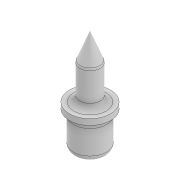
# Autodesk Inventor part: Punta calibración 2
Saved by Autodesk Inventor 2022 (Build 260153000, 153)
## iProperties
Created: 2022-11-17
Part Number: Punta calibración 2
Material: Generic
Document SubType Name: Modeling
Designer: ADMIN
Density: 1 g/cm^3
Appearance: Default
Author: ADMIN
## iProperties of the stored document Punta calibración 2_3DPrint.ipt
Created: 2022-11-17
Part Number: Punta calibración 2_3DPrint
Material: Generic
Document SubType Name: Modeling
Designer: ADMIN
Density: 1 g/cm^3
Appearance: Default
Author: ADMIN
Autodesk Inventor part; units mm, degrees
ref_plane "YZ Plane" through (0, 0, 0) normal (1, 0, 0) x (0, 1, 0)
ref_plane "XZ Plane" through (0, 0, 0) normal (0, 1, 0) x (-1, 0, 0)
ref_plane "XY Plane" through (0, 0, 0) normal (0, 0, 1) x (1, 0, 0)
sketch "Sketch1" plane through (0, 0, 0) normal (0, 1, 0) x (-1, 0, 0)
  circle A0 centre (0, 0) radius 5.6
  dimension "d0" = 11.2
  constraints: 1 centre point, 1 coincident
  measures "d0" diameter of A0
extrude "Extrusion1" add sketch "Sketch1" along normal blind 12
fillet "Fillet1" radius 2 1 edges at (5.6, 0, 0)
sketch "Sketch2" plane through (0, 12, 0) normal (0, 1, 0) x (1, 0, 0)
  circle A0 centre (0, 0) radius 7
  dimension "d4" = 14
  constraints: 1 centre point, 1 coincident
  measures "d4" diameter of A0
extrude "Extrusion2" add sketch "Sketch2" along normal blind 2
sketch "Sketch3" plane through (0, 0, 0) normal (1, 0, 0) x (0, 1, 0)
  line L0 (14, -7) -> (14, 7) projected
  line L1 (12, -7) -> (12, 7) projected
  line L2 (14, 0) -> (35, 0)
  line L3 (35, 0) -> (25.9829, -3.4613)
  line L4 (25.9829, -3.4613) -> (14, -3.4613)
  point P0 (0, 0)
  dimension "d7" = 21
  dimension "d8" = 21
  constraints: 6 end point, 1 horizontal, 1 midpoint, 1 parallel, 1 point on line
  measures "d7" distance of L2.start L2.end
  measures "d8" angle of L3 L2
revolve "Revolution1" add sketch "Sketch3" angle 360 about axis through (0, 14, 0) along (0, 1, 0)
fillet "Fillet2" radius 2 3 edges at (5.6, 12, 0) (0, 14, 3.4613) (0, 25.9829, 3.4613)
body "Solid1"
